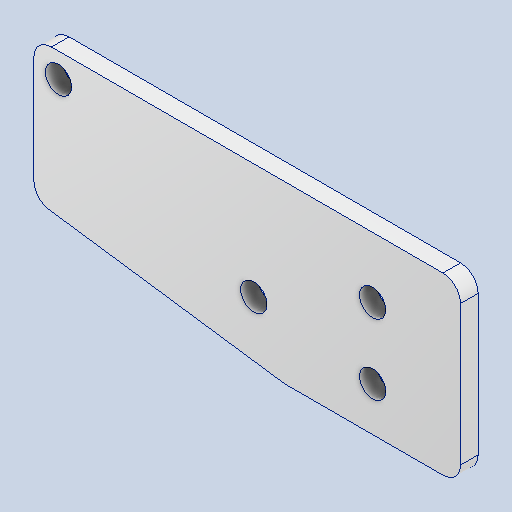
# Autodesk Inventor part: dribl-v1-Plate-12
Saved by Autodesk Inventor 2025.2 (Build 292293000, 293)
## iProperties
Created: 2025-01-15
Part Number: dribl-v1-Plate-12
Material: アルミニウム 6061
Document SubType Name: Modeling
Designer: haruy
Density: 2.7 g/cm^3
Appearance: アルミニウム - フラット
Author: haruy
Autodesk Inventor part; units mm, degrees
ref_plane "YZ Plane" through (0, 0, 0) normal (1, 0, 0) x (0, 1, 0)
ref_plane "XZ Plane" through (0, 0, 0) normal (0, 1, 0) x (-1, 0, 0)
ref_plane "XY Plane" through (0, 0, 0) normal (0, 0, 1) x (1, 0, 0)
sketch "スケッチ1" plane through (0, 0, 0) normal (0, 0, 1) x (1, 0, 0)
  line L0 (203.1661, 661.0271) -> (203.1661, -646.9853)
  line L1 (203.1661, 628.7976) -> (183.1661, 628.7976)
  line L2 (183.1661, 660.9684) -> (183.1661, -646.9853)
  line L3 (183.1661, 25.0147) -> (203.1661, 25.0147)
  line L4 (183.1661, -646.9853) -> (203.1661, -646.9853)
  line L5 (183.1661, 660.9684) -> (203.1661, 661.0271)
  line L6 (168.1661, 612.8976) -> (195.9661, 612.8976)
  line L7 (195.9661, 612.8976) -> (195.9661, 628.7976)
  line L8 (195.9661, 628.7976) -> (168.1661, 628.7976)
  line L9 (168.1661, 628.7976) -> (168.1661, 612.8976)
  circle A0 centre (170.9661, 615.6976) radius 1.5
  circle A1 centre (193.1661, 625.9976) radius 1.5
  circle A2 centre (193.1661, 633.9976) radius 1.5
  line L10 (154.6661, 79.2604) -> (182.4661, 79.2604)
  line L11 (182.4661, 79.2604) -> (182.4661, 63.3604)
  line L12 (182.4661, 63.3604) -> (154.6661, 63.3604)
  line L13 (154.6661, 63.3604) -> (154.6661, 79.2604)
  circle A3 centre (157.4661, 76.4604) radius 1.5
  circle A4 centre (179.6661, 66.1604) radius 1.5
  circle A5 centre (193.1661, 64.3604) radius 1.5
  line L14 (183.1661, 638.9976) -> (203.1661, 638.9976)
  line L15 (195.9661, 612.8976) -> (203.1661, 612.8976)
  line L16 (203.1661, 612.8976) -> (203.1661, 638.9976)
  line L17 (183.1661, 638.9976) -> (168.1661, 628.7976)
  line L18 (183.1661, 59.3604) -> (203.1661, 59.3604)
  line L19 (182.4661, 79.2604) -> (203.1661, 79.2604)
  line L20 (203.1661, 79.2604) -> (203.1661, 59.3604)
  line L21 (183.1661, 59.3604) -> (154.6661, 63.3604)
  circle A6 centre (193.1661, 72.3604) radius 1.5
  point P0 (0, 0)
  point P1 (-212.8828, -214.6519)
  dimension "d0" = 672
  dimension "d1" = 27.8
  dimension "d2" = 15.9
  dimension "d3" = 3
  dimension "d4" = 3
  dimension "d5" = 2.8
  dimension "d6" = 2.8
  dimension "d7" = 2.8
  dimension "d8" = 2.8
  dimension "d9" = 0
  dimension "d10" = 10
  dimension "d11" = 3
  dimension "d12" = 8
  dimension "d13" = 10
  dimension "d14" = 27
  dimension "d15" = 27.8
  dimension "d16" = 15.9
  dimension "d17" = 3
  dimension "d18" = 3
  dimension "d19" = 2.8
  dimension "d20" = 2.8
  dimension "d21" = 2.8
  dimension "d22" = 2.8
  dimension "d24" = 560
  dimension "d25" = 3
  dimension "d27" = 10
  dimension "d28" = 5
  dimension "d29" = 5
  dimension "d33" = 20
  dimension "d34" = 203.1661
  dimension "d39" = 3.5
  dimension "d40" = 3
  dimension "d41" = 10
  dimension "d42" = 8
  dimension "d43" = 4
  constraints: 44 end point, 10 point on line, 7 centre point, 7 perpendicular, 5 horizontal, 4 parallel
  measures "d0" distance between parallel lines of L4 L3
  measures "d1" distance of L8.end L7.end
  measures "d2" distance of L7.end L6.end
  measures "d3" diameter of A0
  measures "d4" diameter of A1
  measures "d5" distance from line of A0.centre L6
  measures "d6" distance from line of A0.centre L9
  measures "d7" distance from line of A1.centre L8
  measures "d8" distance from line of L7 A1.centre
  measures "d9" distance between parallel lines of L1 L8
  measures "d10" distance from line of A1.centre L2
  measures "d11" diameter of A2
  measures "d12" distance of A1.centre A2.centre
  measures "d13" distance from line of L2 A2.centre
  measures "d14" distance from line of A2.centre L5
  measures "d15" distance of L11.end L12.end
  measures "d16" distance of L10.end L11.end
  measures "d17" diameter of A3
  measures "d18" diameter of A4
  measures "d19" distance from line of A3.centre L10
  measures "d20" distance from line of A3.centre L13
  measures "d21" distance from line of A4.centre L12
  measures "d22" distance from line of L11 A4.centre
  measures "d24" distance of A1.centre A4.centre
  measures "d25" diameter of A5
  measures "d27" distance from line of A5.centre L2
  measures "d28" distance from line of A2.centre L14
  measures "d29" distance from line of A5.centre L18
  measures "d33" distance between parallel lines of L0 L2
  measures "d34" distance from line of L0 point (0, 0)
  measures "d39" distance from line of L2 A4.centre
  measures "d40" diameter of A6
  measures "d41" distance from line of L0 A6.centre
  measures "d42" distance of A5.centre A6.centre
  measures "d43" distance between parallel lines of L18 L12
extrude "押し出し1" add sketch "スケッチ1" against normal blind 2 contours L0 L18 L2 L19 | L2 L21 L12 L11 L19 | L11 L12 L13 L10
fillet "フィレット1" radius 2 5 edges at (154.6661, 79.2604, -1) (154.6661, 63.3604, -1) (183.1661, 59.3604, -1) (203.1661, 59.3604, -1) (203.1661, 79.2604, -1)
equation "\"d6\" = d5"
equation "\"d7\" = d5"
equation "\"d8\" = d5"
equation "\"d20\" = d19"
equation "\"d21\" = d19"
equation "\"d22\" = d19"
